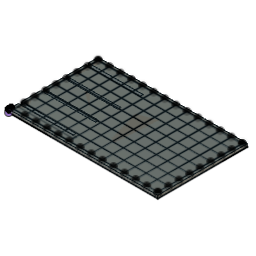
Universal Spoilboard (Autodesk Fusion 360 design; units mm, degrees)
Autodesk Fusion 360 part; units mm, degrees
sketch "Half Spoilboard" plane through (0, 0, 0) normal (0, 0, 1) x (1, 0, 0)
  line L0 (0, 0) -> (0, 22.5) construction
  line L1 (0, 19.5) -> (110, 19.5)
  line L2 (110, 19.5) -> (110, 25.5)
  line L3 (110, 25.5) -> (0, 25.5)
  line L4 (0, 25.5) -> (0, 19.5)
  line L5 (0, 0) -> (300, 0)
  line L6 (300, 0) -> (300, 180)
  line L7 (300, 180) -> (0, 180)
  line L8 (0, 180) -> (0, 0)
  dimension "d10" = 22.5
  dimension "d11" = 6
  dimension "d12" = 110
  dimension "d13" = 300
  dimension "d14" = 180
  constraint coincident L0.start L5.start
  constraint vertical L0
  constraint horizontal L1
  constraint vertical L2
  constraint horizontal L3
  constraint vertical L4
  constraint midpoint L0.end L4
  constraint horizontal L5
  constraint vertical L6
  constraint horizontal L7
  constraint vertical L8
  measures "d10" distance of L0.start L0.end
  measures "d11" distance of L1.end L2.end
  measures "d12" distance of L2.end L3.end
  measures "d13" distance of L0.start L5.end
  measures "d14" distance of L0.start L7.end
extrude "Extrude1" add sketch "Half Spoilboard" along normal blind 6 contours L1 L2 L3 L5 L6 L7 L8
pattern_linear "R-Pattern1" count 4 spacing 45 along (0, 1, 0) of 3 faces at (110, 21.5, 2) (36.6667, 19.5, 2) (73.3333, 25.5, 2)
sketch "Sketch3" plane through (0, 0, 6) normal (0, 0, 1) x (-1, 0, 0)
  line L0 (-110, -154.5) -> (0, -154.5)
  line L1 (0, -154.5) -> (0, -115.5)
  line L2 (0, -115.5) -> (-110, -115.5)
  line L3 (-110, -115.5) -> (-110, -109.5)
  line L4 (-110, -109.5) -> (0, -109.5)
  line L5 (0, -109.5) -> (0, -70.5)
  line L6 (0, -70.5) -> (-110, -70.5)
  line L7 (-110, -70.5) -> (-110, -64.5)
  line L8 (-110, -64.5) -> (0, -64.5)
  line L9 (0, -64.5) -> (0, -25.5)
  line L10 (0, -25.5) -> (-110, -25.5)
  line L11 (-110, -25.5) -> (-110, -19.5)
  line L12 (-110, -19.5) -> (0, -19.5)
  line L13 (0, -19.5) -> (0, 0)
  line L14 (0, 0) -> (-300, 0)
  line L15 (-300, 0) -> (-300, -180)
  line L16 (-300, -180) -> (0, -180)
  line L17 (0, -180) -> (0, -160.5)
  line L18 (0, -160.5) -> (-110, -160.5)
  line L19 (-110, -160.5) -> (-110, -154.5)
  line L20 (0, 0) -> (0, -5) construction
  line L21 (-5, -5) -> (0, -5) construction
  line L22 (-5, -5) -> (-295, -5)
  line L23 (-5, -5) -> (-5, -175)
  line L24 (-5, -26.25) -> (-295, -26.25)
  line L25 (-5, -47.5) -> (-295, -47.5)
  line L26 (-5, -68.75) -> (-295, -68.75)
  line L27 (-5, -90) -> (-295, -90)
  line L28 (-5, -111.25) -> (-295, -111.25)
  line L29 (-5, -132.5) -> (-295, -132.5)
  line L30 (-5, -153.75) -> (-295, -153.75)
  line L31 (-27.3077, -5) -> (-27.3077, -175)
  line L32 (-49.6154, -5) -> (-49.6154, -175)
  line L33 (-71.9231, -5) -> (-71.9231, -175)
  line L34 (-94.2308, -5) -> (-94.2308, -175)
  line L35 (-116.5385, -5) -> (-116.5385, -175)
  line L36 (-138.8462, -5) -> (-138.8462, -175)
  line L37 (-161.1538, -5) -> (-161.1538, -175)
  line L38 (-183.4615, -5) -> (-183.4615, -175)
  line L39 (-205.7692, -5) -> (-205.7692, -175)
  line L40 (-228.0769, -5) -> (-228.0769, -175)
  line L41 (-250.3846, -5) -> (-250.3846, -175)
  line L42 (-272.6923, -5) -> (-272.6923, -175)
  line L43 (-5, -175) -> (-295, -175)
  line L44 (-295, -5) -> (-295, -175)
  dimension "d46" = 5
  dimension "d47" = 5
  dimension "d48" = 290
  dimension "d49" = 170
  dimension "d52" = 0
  dimension "d57" = 0
  constraint coincident L13.end L14.start
  constraint coincident L13 L20.end
  constraint perpendicular L14 L20
  constraint perpendicular L13 L21
  constraint parallel L21 L22
  constraint perpendicular L8 L23
  measures "d46" distance of L20.end L21.start
  measures "d47" distance of L13.end L20.end
  measures "d48" distance of L21.start L22.end
  measures "d49" distance of L21.start L23.end
equation "bedX = 300 mm" comment "Dimension of the bed in X (Width)"
equation "bedY = 180 mm" comment "Dimension of the bed in Y (Height)"
equation "spoilboardThickness = 6 mm" comment "Thickness of the Spoilboard stock"
equation "slots = 4" comment "Number of slots in the bed"
equation "slotY = 6 mm" comment "Height of each slot in the spoilboard (Y)"
equation "minStockX = 80 mm" comment "Width of the uncut area in the middle of the spoilboard"
equation "slotX = ( bedX - minStockX ) / 2" comment "Length of each slot from the edge of the stock (X)"
equation "slotSpacing = bedY / slots" comment "Distance between centrelines of the slots on the Y axis"
equation "slotEdgeSpacing = slotSpacing / 2" comment "Distance between the front edge of the bed and the first slot centreline"
equation "d10 = slotEdgeSpacing"
equation "d11 = slotY"
equation "d12 = slotX"
equation "d13 = bedX"
equation "d14 = bedY"
equation "d15 = spoilboardThickness"
equation "d17 = slots"
equation "d19 = slotSpacing"
equation "gridXLines = 14" comment "Number of lines to be engraved vertically along the X axis"
equation "XFromEdge = 5 mm" comment "Distance from the left of the bed to the cutting area"
equation "gridYLines = 9" comment "Number of lines to be engraved horizontally along the Y axis"
equation "YFromEdge = 5 mm" comment "Distance from the front of the bed to the cutting area"
equation "cutX = 290 mm" comment "Width of the cutting area (X)"
equation "cutY = 170 mm" comment "Depth of the cutting area (Y)"
equation "d46 = XFromEdge"
equation "d47 = YFromEdge"
equation "d48 = cutX"
equation "d49 = cutY"
equation "d51 = gridYLines"
equation "d53 = -cutY"
equation "d54 = gridXLines"
equation "d56 = -cutX"
named bodies: "Half Spoilboard"
